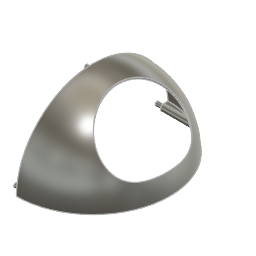
cabeza parte delantera (Autodesk Fusion 360 design; units mm, degrees)
part number: 2026-06-26-00-22-46-381
Autodesk Fusion 360 part; units mm, degrees
note: some values were not read from the file. Chosen so that the rebuilt part matches the saved one: which pieces of a blend or face edit are solid.
sketch "Boceto1" plane through (0, 0, 0) normal (0, 1, 0) x (1, 0, 0)
  line L0 (0, 57.5) -> (0, -57.5)
  arc A0 (0, -57.5) -> (0, 57.5) centre (0, 0) ccw
  arc A1 (0, -56.5) -> (0, 56.5) centre (0, 0) ccw
  ellipse E0 centre (37.1476, 0.0888) end of major axis (37.1476, 32) minor radius 18.4234
  line L1 (37.1476, -31.8224) -> (37.1476, 32) construction
  line L2 (55.571, 0.0888) -> (18.7242, 0.0888) construction
  dimension "d1" = 115
  dimension "d2" = 56.5
  constraint coincident A0.centre A1.centre
  constraint vertical L0
  constraint coincident L0 A1.start
  constraint coincident E0 L1.start
  constraint coincident E0 L1.end
  constraint coincident E0 L2.start
  constraint coincident E0 L2.end
  constraint vertical L1
  measures "d1" diameter of A0
  measures "d2" radius of A1
revolve "Revolución1" add sketch "Boceto1" angle 90 about axis through (0, 0, -57.5) along (0, 0, 1) contours L0 A0 A1 makes body 1
extrude "Extruir1" cut sketch "Boceto1" along normal blind 70 contours E0 bodies 1
sketch "Boceto2" plane through (0, 0, 0) normal (-1, 0, 0) x (0, 0, 1)
  arc A0 (57.5, 0) -> (-57.5, 0) centre (0, 0) ccw
  line L0 (-57.5, 0) -> (-56.5, 0)
  arc A1 (56.5, 0) -> (-56.5, 0) centre (0, 0) ccw
  line L1 (56.5, 0) -> (57.5, 0)
  line L2 (-56.5, 0) -> (-53, 0)
  line L3 (-56.2783, 5) -> (-53, 5)
  arc A2 (-53, 0) -> (-53, 5) centre (-53, 2.5) ccw
  circle A3 centre (-53, 2.5) radius 1.55
  line L4 (56.5, 0) -> (53, 0)
  line L5 (56.2783, 5) -> (53, 5)
  arc A4 (53, 5) -> (53, 0) centre (53, 2.5) ccw
  circle A5 centre (53, 2.5) radius 1.55
  line L6 (-2.5, 56.4447) -> (-2.5, 53)
  line L7 (2.5, 56.4447) -> (2.5, 53)
  arc A6 (-2.5, 53) -> (2.5, 53) centre (0, 53) ccw
  circle A7 centre (0, 53) radius 1.55
  dimension "d6" = 3.5
  dimension "d8" = 3.1
  dimension "d9" = 3.5
  dimension "d10" = 3.1
  dimension "d14" = 3.1
  constraint coincident L0.end A1.end
  constraint parallel L0 L2
  constraint concentric A2 A3
  constraint coincident A1 L3.start
  constraint coincident A1.start L1.start
  constraint parallel L1 L4
  constraint tangent L5 A4
  constraint concentric A4 A5
  constraint coincident A1 L5.start
  constraint tangent L6 A6
  constraint concentric A6 A7
  constraint coincident A1 L6.start
  constraint coincident A1 L7.start
  measures "d6" distance of L0.end L2.end
  measures "d8" diameter of A3
  measures "d9" distance of A1.start L4.end
  measures "d10" diameter of A5
  measures "d14" diameter of A7
extrude "Extruir2" add sketch "Boceto2" against normal blind 45 contours A1 L4 L5 A4 | A1 L2 L3 A2 bodies 1
delete_face "SuprimirCaras1" 1 faces at (22.1181, 2.7803, 56.4316) on bodies 1
delete_face "SuprimirCaras2" 1 faces at (22.1181, 2.7803, -56.4316) on bodies 1
extrude "Extruir3" add sketch "Boceto2" along normal blind 5 and the other way blind 35 contours A3 | A5 bodies 1
delete_face "SuprimirCaras3" 1 faces at (27.3707, 3.8704, 52.2757) on bodies 1
delete_face "SuprimirCaras4" 1 faces at (27.1332, 0.9989, -52.6139) on bodies 1
extrude "Extruir4" add sketch "Boceto2" against normal blind 5 separate body contours A7 makes body 2
extrude "Extruir5" add sketch "Boceto2" against normal blind 5 contours A1 L6 L7 A6 bodies 1 2
extrude "Extruir6" add sketch "Boceto2" along normal blind 5 contours A7 bodies 1
revolve "Revolución2" add sketch "Boceto1" angle 90 about axis through (0, 0, -57.5) along (0, 0, 1) contours L0 A0 A1 bodies 1
extrude "Extruir7" cut sketch "Boceto1" along normal blind 65 contours E0 bodies 1
delete_face "SuprimirCaras5" 1 faces at (5, 54.0907, -0.2779) on bodies 1
extrude "Extruir8" add sketch "Boceto2" against normal blind 10 separate body contours A7 makes body 3
extrude "Extruir9" add sketch "Boceto2" against normal blind 10 contours A1 L6 L7 A6 bodies 1 3
extrude "Extruir10" add sketch "Boceto2" along normal blind 5 contours A7 bodies 1
